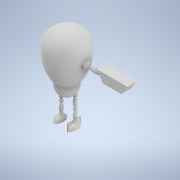
# Autodesk Inventor part: Model-robot
Saved by Autodesk Inventor 2020 (Build 240168000, 168)
## iProperties
Created: 2019-10-24
Part Number: Model-robot
Material: Generic
Document SubType Name: Modeling
Designer: Victor
Density: 1 g/cm^3
Appearance: Default
Author: Victor
Autodesk Inventor part; units mm, degrees
ref_plane "XZ Plane" through (0, 0, 0) normal (0, 1, 0) x (-1, 0, 0)
ref_plane "XY Plane" through (0, 0, 0) normal (0, 0, 1) x (1, 0, 0)
sketch "Sketch1" plane through (0, 0, 0) normal (0, 0, 1) x (1, 0, 0)
  ellipse E0 centre (15, 0) end of major axis (15, 13) minor radius 7
  line L0 (0, 13.131441) -> (0, -13.043697)
  ellipse E1 centre (-15, 0) end of major axis (-15, 13) minor radius 7
  point P0 (0, 0)
  dimension "d0" = 13
  dimension "d1" = 7
  dimension "d2" = 15
  constraints: 2 end point, 2 vertical, 1 symmetric about line, 4 other
  measures "d2" distance of point (15, 0) point (0, 0)
extrude "Extrusion1" add sketch "Sketch1" along normal blind 10
sketch "Sketch2" plane through (0, 0, 0) normal (1, 0, 0) x (0, 1, 0)
  line L0 (13, 10) -> (-13, 10)
  line L1 (13, 0) -> (-13, 0)
  arc A0 (0, 10) -> (-13, 0) centre (-0.500799, -2.798961) ccw
  line L2 (0, 10) -> (7, 10)
  arc A1 (13, 0) -> (7, 10) centre (1.877748, 0.126649) ccw
  line L3 (13, 0) -> (-13, 0)
  line L4 (13, 10) -> (-13, 10)
  line L5 (-13, 0) -> (-13, 10)
  line L6 (-13, 10) -> (-1.001598, 10)
  line L7 (7, 10) -> (13, 10)
  line L8 (13, 10) -> (13, 0)
  point P0 (0, 0)
  point P1 (13, 0.253297)
  point P2 (-1.001598, 10)
  dimension "d5" = 7
  constraints: 10 end point, 5 point on circle, 2 centre point, 2 point on line, 1 collinear, 1 midpoint, 1 perpendicular, 1 vertical
  measures "d5" distance of L2.start L2.end
sketch "Sketch2 outline for Extrusion2" plane through (0, 0, 0) normal (1, 0, 0) x (0, 1, 0)
  line L0 (13, 0.253297) -> (13, 10)
  arc A0 (7, 10) -> (13, 0.253297) centre (1.877748, 0.126649) cw
  line L1 (13, 10) -> (7, 10)
  line L2 (-13, 10) -> (-13, 0)
  line L3 (-1.001598, 10) -> (-13, 10)
  arc A1 (-13, 0) -> (-1.001598, 10) centre (-0.500799, -2.798961) cw
extrude "Extrusion2" cut sketch "Sketch2 outline for Extrusion2" along normal mid plane 50
sketch "Sketch3" plane through (0, 0, 0) normal (0, 1, 0) x (-1, 0, 0)
  line L0 (22, 0) -> (8, 0)
  arc A0 (22, 0) -> (19, 10) centre (5.473116, 0.491935) ccw
  line L1 (15, 0) -> (15, 10)
  line L2 (22, 10) -> (20.898551, 10)
  line L3 (19, 10) -> (22, 10)
  line L4 (22, 10) -> (22, 0)
  arc A1 (11, 10) -> (8, 0) centre (24.526884, 0.491935) ccw
  line L5 (11, 10) -> (8, 10)
  line L6 (8, 10) -> (8, 0)
  line L7 (0, 16.989646) -> (0, -10.119473)
  line L8 (-22, 0) -> (-8, 0)
  arc A2 (-19, 10) -> (-22, 0) centre (-5.473116, 0.491935) ccw
  line L9 (-15, 0) -> (-15, 10)
  line L10 (-22, 10) -> (-20.898551, 10)
  line L11 (-19, 10) -> (-22, 10)
  line L12 (-22, 10) -> (-22, 0)
  arc A3 (-8, 0) -> (-11, 10) centre (-24.526884, 0.491935) ccw
  line L13 (-11, 10) -> (-8, 10)
  line L14 (-8, 10) -> (-8, 0)
  point P0 (0, 0)
  point P1 (21.979193, 10)
  point P2 (-21.979193, 10)
  point P3 (-22, 0.98387)
  point P4 (-8, 0.98387)
  point P5 (22, 0.98387)
  point P6 (8, 0.98387)
  dimension "d9" = 3
  constraints: 26 end point, 20 symmetric about line, 12 point on circle, 4 centre point, 1 horizontal, 1 perpendicular, 1 vertical, 3 other
  measures "d9" horizontal distance of L3.start L0.start
extrude "Extrusion3" cut sketch "Sketch3" along normal mid plane 50 contours A0 L3 L2 L4 | A1 L6 L5 | A2 L12 L10 L11 | A3 L13 L14
sketch "Sketch4" plane through (0, 0, 10) normal (0, 0, 1) x (1, 0, 0)
  arc A0 (15, 7) -> (15, -1) centre (15, 3) ccw
  line L0 (11, -1.001598) -> (19, -1.001598)
  line L1 (15, -1.001598) -> (15, 7)
  line L2 (19, 7) -> (11, 7)
  point P0 (0, 0)
  constraints: 3 midpoint, 2 end point, 2 point on circle, 1 centre point, 1 point on line
revolve "Revolution1" add sketch "Sketch4" angle 360 about axis through (15, -1.001598, 10) along (0, 1, 0)
ref_plane "Work Plane1" through (15, 0, 0) normal (1, 0, 0) x (0, 1, 0)
sketch "Sketch5" plane through (15, 0, 0) normal (1, 0, 0) x (0, 1, 0)
  line L0 (-1.001598, 10) -> (7, 10)
  line L1 (2.999201, 10) -> (2.999201, 35)
  line L2 (3, 10) -> (7, 10)
  arc A0 (2.999201, 35) -> (3, 10) centre (20.524401, 22.50056) ccw
  point P0 (0, 0)
  point P1 (2.999201, 10.00112)
  dimension "d16" = 25
  dimension "d20" = 21.526
  constraints: 2 end point, 2 point on circle, 1 centre point, 1 midpoint, 1 vertical
  measures "d16" distance of L1.start L1.end
  measures "d20" radius of A0
revolve "Revolution2" add sketch "Sketch5" angle 360 about axis through (15, 2.999201, 10) along (0, 0, 1)
sketch "Sketch6" plane through (15, 0, 0) normal (1, 0, 0) x (0, 1, 0)
  arc A0 (2.999201, 35) -> (0.989728, 13.458151) centre (20.524401, 22.50056) ccw
  circle A1 centre (2.999201, 35) radius 4
  line L0 (2.999201, 39) -> (2.999201, 31)
  point P0 (0, 0)
  dimension "d18" = 8
  constraints: 3 point on circle, 2 end point, 1 centre point, 1 vertical
  measures "d18" diameter of A1
revolve "Revolution3" add sketch "Sketch6" angle 360 about axis through (15, 2.999201, 39) along (0, 0, -1) contours L0 A1
sketch "Sketch7" plane through (15, 0, 0) normal (1, 0, 0) x (0, 1, 0)
  arc A0 (2.999201, 60) -> (2.999201, 35) centre (20.524003, 47.5) ccw
  line L0 (2.999201, 60) -> (2.999201, 35)
  point P0 (0, 0)
  point P1 (-1.031809, 60)
  dimension "d21" = 25
  dimension "d22" = 21.526
  constraints: 2 end point, 2 point on circle, 1 centre point, 1 vertical
  measures "d21" distance of L0.end L0.start
  measures "d22" radius of A0
revolve "Revolution4" add sketch "Sketch7" angle 360 about axis through (15, 2.999201, 60) along (0, 0, -1)
sketch "Sketch8" plane through (15, 0, 0) normal (1, 0, 0) x (0, 1, 0)
  arc A0 (2.999201, 60) -> (0.989039, 38.458215) centre (20.524003, 47.5) ccw
  circle A1 centre (2.999201, 60) radius 4
  line L0 (2.999201, 64) -> (2.999201, 56)
  point P0 (0, 0)
  dimension "d24" = 8
  constraints: 3 point on circle, 2 end point, 1 centre point, 1 vertical
  measures "d24" diameter of A1
revolve "Revolution5" add sketch "Sketch8" angle 360 about axis through (15, 2.999201, 64) along (0, 0, -1) contours L0 A1
sketch "Sketch9" plane through (0, 0, 0) normal (1, 0, 0) x (0, 1, 0)
  circle A0 centre (0, 75) radius 21.00893
  line L0 (0, 75) -> (21.00893, 75)
  line L1 (0, 75) -> (0, 53.99107)
  arc A1 (0.989039, 56.541785) -> (0.989039, 38.458215) centre (20.524003, 47.5) ccw
  point P0 (0, 0)
  constraints: 4 end point, 3 point on circle, 1 centre point, 1 horizontal
revolve "Revolution6" add sketch "Sketch9" angle 360 about axis through (0, 0, 75) along (0, 0, -1) picked at (13.830374, 73.441691) contours A0 L1 L0
pattern_linear "Rectangular Pattern1" count 2 spacing 30 along (-1, 0, 0) of "Revolution4", "Revolution3", "Revolution5", "Revolution2", "Revolution1"
sketch "Sketch11" plane through (0, 0, 0) normal (0, 1, 0) x (-1, 0, 0)
  line L0 (-21.00893, 75) -> (21.00893, 75)
  line L1 (0, 75) -> (0, 87)
  line L2 (0, 87) -> (-21.00893, 87)
  line L3 (0, 75) -> (-21.00893, 75)
  arc A0 (-21.00893, 75) -> (-21.00893, 87) centre (-35.841327, 81) ccw
  point P0 (0, 0)
  dimension "d30" = 12
  dimension "d31" = 16
  dimension "d32" = 35.84133
  constraints: 6 end point, 2 point on circle, 1 centre point, 1 horizontal, 1 midpoint, 1 perpendicular, 1 vertical
  measures "d30" distance of L1.start L1.end
  measures "d31" radius of A0
  measures "d32" horizontal distance of L1.start A0.centre
revolve "Revolution7" add sketch "Sketch11" angle 360 about axis through (0, 0, 75) along (0, 0, 1)
sketch "Sketch13" plane through (0, 0, 0) normal (0, 1, 0) x (-1, 0, 0)
  line L0 (21.00893, 87) -> (-21.00893, 87)
  line L1 (0, 87) -> (-25, 87)
  line L2 (0, 176.999187) -> (0, 87)
  arc A0 (0, 176.999187) -> (-11.880257, 177.163489) centre (-6.554203, 132.679178) ccw
  arc A1 (-40.159828, 148.063755) -> (-25, 87) centre (55.431258, 139.381733) ccw
  arc A2 (-11.880257, 177.163489) -> (-40.159828, 148.063755) centre (-8.046975, 145.147118) ccw
  point P0 (0, 0)
  point P1 (-48.551096, 142.44381)
  point P2 (-38.302597, 164.290257)
  point P3 (-30.103423, 170.440665)
  dimension "d35" = 25
  constraints: 6 point on circle, 4 end point, 3 centre point, 2 tangent, 1 collinear, 1 midpoint, 1 vertical
  measures "d35" distance of L1.start L1.end
revolve "Revolution8" add sketch "Sketch13" angle 360 about axis through (0, 0, 176.999187) along (0, 0, -1)
sketch "Sketch14" plane through (0, 0, 0) normal (0, 1, 0) x (-1, 0, 0)
  arc A0 (-40.159828, 148.063755) -> (-25, 87) centre (55.431258, 139.381733) ccw
  circle A1 centre (-40.159828, 130.699711) radius 8.75
  line L0 (-40.159828, 130.699711) -> (-40.159828, 121.949711)
  line L1 (-40.159828, 130.699711) -> (-40.159828, 139.449711)
  point P0 (0, 0)
  point P1 (-40.55327, 139.440861)
  dimension "d38" = 17.5
  constraints: 4 end point, 3 point on circle, 1 centre point, 1 point on line, 1 vertical
  measures "d38" diameter of A1
revolve "Revolution9" add sketch "Sketch14" angle 360 about axis through (40.159828, 0, 130.699711) along (0, 0, -1) picked at (-42.987776, 132.627862) contours A0 L0 A1
sketch "Sketch15" plane through (0, 0, 0) normal (0, 1, 0) x (-1, 0, 0)
  line L0 (-42, 130.699711) -> (-82, 130.699711)
  arc A0 (-42, 130.699711) -> (-82, 130.699711) centre (-62, 90.506252) ccw
  point P0 (0, 0)
  dimension "d44" = 40
  dimension "d45" = 42
  constraints: 2 end point, 2 point on circle, 1 centre point, 1 horizontal
  measures "d44" distance of L0.start L0.end
  measures "d45" horizontal distance of L0.start point (0, 0)
revolve "Revolution10" add sketch "Sketch15" angle 360 about axis through (42, 0, 130.699711) along (1, 0, 0)
sketch "Sketch16" plane through (0, 0, 0) normal (0, 1, 0) x (-1, 0, 0)
  arc A0 (-48.506705, 133.324999) -> (-82, 130.699711) centre (-62, 90.506252) ccw
  circle A1 centre (-82, 130.699711) radius 6.25
  line L0 (-82, 136.949711) -> (-82, 124.449711)
  point P0 (0, 0)
  dimension "d46" = 12.5
  constraints: 3 point on circle, 2 end point, 1 centre point, 1 vertical
  measures "d46" diameter of A1
revolve "Revolution12" add sketch "Sketch16" angle 360 about axis through (82, 0, 136.949711) along (0, 0, -1) contours L0 A1
sketch "Sketch17" plane through (0, 0, 0) normal (0, 1, 0) x (-1, 0, 0)
  arc A0 (-76.224217, 133.087771) -> (-76.224217, 128.31165) centre (-82, 130.699711) ccw
  line L0 (-82, 124.449711) -> (-87.5, 124.449711)
  line L1 (-87.5, 124.449711) -> (-75.064213, 144.449711)
  line L2 (-75.064213, 144.449711) -> (-105.064213, 144.449711)
  line L3 (-87.5, 124.449711) -> (-127.5, 124.449711)
  line L4 (-105.064213, 144.449711) -> (-140.064213, 144.449711)
  line L5 (-127.5, 124.449711) -> (-140.064213, 144.449711)
  point P0 (0, 0)
  point P1 (-86.383758, 126.24492)
  point P2 (-79.943937, 136.601838)
  dimension "d48" = 5.5
  dimension "d49" = 20
  dimension "d50" = 140.02091
  dimension "d51" = 30
  dimension "d52" = 40
  dimension "d53" = 35
  constraints: 12 end point, 4 horizontal, 1 point on circle, 1 tangent
  measures "d48" distance of L0.start L0.end
  measures "d49" vertical distance of L0.end L1.end
  measures "d50" distance from line of point (0, 0) L1
  measures "d51" distance of L1.end L2.end
  measures "d52" distance of L0.end L3.end
  measures "d53" distance of L2.end L4.end
extrude "Extrusion4" add sketch "Sketch17" along normal mid plane 20 contours L1 A0 | A0 L1 L3 L5 L4 L2
body "Solid1"
